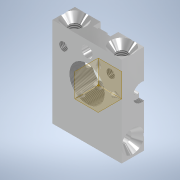
# Autodesk Inventor part: CuvetteHolderBody
Saved by Autodesk Inventor 2022 (Build 260153000, 153)
## iProperties
Created: 2021-04-01
Part Number: CuvetteHolderBody
Material: Aluminum 6061
Document SubType Name: Modeling
Designer: wilso
Density: 2.7 g/cm^3
Appearance: Aluminum - Flat
Author: wilso
Autodesk Inventor part; units mm, degrees
ref_plane "YZ Plane" through (0, 0, 0) normal (1, 0, 0) x (0, 1, 0)
ref_plane "XZ Plane" through (0, 0, 0) normal (0, 1, 0) x (-1, 0, 0)
ref_plane "XY Plane" through (0, 0, 0) normal (0, 0, 1) x (1, 0, 0)
sketch "Sketch1" plane through (0, 0, 0) normal (0, 1, 0) x (-1, 0, 0)
  line L0 (0, 0) -> (50, 0)
  line L1 (50, 0) -> (50, -16.15)
  line L2 (50, -16.15) -> (0, -16.15)
  line L3 (0, -16.15) -> (0, 0)
  dimension "d0" = 50
  dimension "d1" = 16.15
  constraints: 8 end point, 2 parallel, 1 horizontal, 1 perpendicular
  measures "d0" distance of L1.end L2.end
  measures "d1" distance of L0.end L1.end
extrude "Extrusion1" add sketch "Sketch1" along normal blind 65
sketch "Sketch2" plane through (0, 65, 0) normal (0, 1, 0) x (1, 0, 0)
  line L0 (-50, 0) -> (0, 0) projected
  line L1 (-50, 16.15) -> (-50, 0) projected
  line L2 (0, 0) -> (0, 16.15) projected
  line L3 (0, 16.15) -> (-50, 16.15) projected
  point P0 (-42.0625, 8.075)
  point P1 (-7.9375, 8.075)
  dimension "d11" = 8.075
  dimension "d12" = 7.9375
  dimension "d13" = 8.075
  dimension "d14" = 7.9375
  dimension "d87" = 16.15
  measures "d11" distance from line of L0 point (-42.062, 8.075)
  measures "d12" distance from line of L1 point (-42.062, 8.075)
  measures "d13" distance from line of L0 point (-7.938, 8.075)
  measures "d14" distance from line of L2 point (-7.938, 8.075)
  measures "d87" distance between parallel lines of L0 L3
hole "Hole1" at (-42.0625, 65, -8.075) at (-7.9375, 65, -8.075) direction (0, -1, 0) diameter 6.35 depth 55 tip angle 118 countersink diameter 16.5 countersink angle 82
sketch "Sketch3" plane through (0, 65, 0) normal (0, 1, 0) x (1, 0, 0)
  line L0 (0, 16.15) -> (-50, 16.15) projected
  line L1 (-18.65, 16.15) -> (-18.65, 10.65)
  line L2 (-18.65, 10.65) -> (-21.825, 10.65)
  line L3 (-21.825, 10.65) -> (-21.825, 11.65)
  line L4 (-21.825, 11.65) -> (-28.175, 11.65)
  line L5 (-28.175, 11.65) -> (-28.175, 10.65)
  line L6 (-28.175, 10.65) -> (-31.35, 10.65)
  line L7 (-31.35, 10.65) -> (-31.35, 16.15)
  point P0 (0, 0)
  dimension "d15" = 5.5
  dimension "d16" = 3.175
  dimension "d17" = 1
  dimension "d18" = 3.175
  dimension "d19" = 6.35
  dimension "d21" = 18.65
  constraints: 14 end point, 6 perpendicular, 4 point on line
  measures "d15" distance of L1.start L1.end
  measures "d16" distance of L1.end L2.end
  measures "d17" distance of L2.end L3.end
  measures "d18" distance of L5.end L6.end
  measures "d19" distance of L3.end L4.end
  measures "d21" distance of L0.end L7.end
extrude "Extrusion2" cut sketch "Sketch3" against normal blind 25
sketch "Sketch4" plane through (-50, 0, 0) normal (0, 0, 1) x (1, 0, 0)
  line L0 (0, 65) -> (50, 65) projected
  line L1 (0, 0) -> (0, 65) projected
  point P0 (50, 0)
  point P1 (25, 37.5)
  dimension "d24" = 27.5
  dimension "d43" = 25
  measures "d24" distance from line of L0 point (25, 37.5)
  measures "d43" distance from line of L1 point (25, 37.5)
hole "Hole2" at (-25, 37.5, 0) direction (0, 0, -1) diameter 25.4 depth 55
thread "Thread1" size "1-32 UN" class "2B" standard "ANSI Unified Screw Threads" full length
sketch "Sketch5" plane through (0, 0, 0) normal (1, 0, 0) x (0, 0, -1)
  line L0 (0, 0) -> (16.15, 0) projected
  line L1 (0, 0) -> (0, 65) projected
  line L2 (16.15, 0) -> (16.15, 65) projected
  point P0 (8.075, 10)
  dimension "d34" = 10
  dimension "d35" = 8.075
  dimension "d88" = 16.15
  measures "d34" distance from line of L0 point (8.075, 10)
  measures "d35" distance from line of L1 point (8.075, 10)
  measures "d88" distance between parallel lines of L1 L2
hole "Hole3" at (0, 10, -8.075) direction (-1, 0, 0) diameter 6.35 depth 45 tip angle 118 countersink diameter 16.5 countersink angle 82
sketch "Sketch6" plane through (-50, 0, 0) normal (0, 0, 1) x (1, 0, 0)
  line L0 (50, 0) -> (50, 65) projected
  line L1 (0, 65) -> (50, 65) projected
  point P0 (25, 57.5)
  dimension "d44" = 25
  dimension "d45" = 7.5
  measures "d44" distance from line of L0 point (25, 57.5)
  measures "d45" distance from line of L1 point (25, 57.5)
hole "Hole4" at (-25, 57.5, 0) direction (0, 0, -1) diameter 7.9375 depth 10.15 tip angle 118
sketch "Sketch7" plane through (-50, 0, -16.15) normal (-1, 0, 0) x (0, 0, 1)
  line L0 (0, 24.8) -> (0, 48.4985) projected
  line L1 (0, 37.5) -> (1.75, 37.5)
  line L2 (16.15, 0) -> (0, 0) projected
  circle A0 centre (1.75, 37.5) radius 3.175
  circle A1 centre (1.75, 37.5) radius 6.35
  dimension "d53" = 1.75
  dimension "d69" = 37.5
  dimension "d70" = 1.75
  dimension "d71" = 6.35
  dimension "d72" = 12.7
  constraints: 2 centre point, 2 coincident, 2 end point, 1 horizontal
  measures "d53" distance of L1.start L1.end
  measures "d69" distance from line of L2 L1.end
  measures "d70" distance from line of L0 L1.end
  measures "d71" diameter of A0
  measures "d72" diameter of A1
extrude "Extrusion6" cut sketch "Sketch7" against normal blind 60 contours A0 L0 | L0 A0
extrude "Extrusion7" cut sketch "Sketch7" against normal blind 3.5
sketch "Sketch9" plane through (0, 0, 0) normal (1, 0, 0) x (0, 0, -1)
  circle A0 centre (14.4, 37.5) radius 6.35
  line L0 (16.15, 0) -> (16.15, 34.8508) projected
  line L1 (0, 0) -> (16.15, 0) projected
  dimension "d77" = 12.7
  dimension "d78" = 1.75
  dimension "d79" = 37.5
  constraints: 1 centre point
  measures "d77" diameter of A0
  measures "d78" distance from line of L0 A0.centre
  measures "d79" distance from line of L1 A0.centre
extrude "Extrusion8" cut sketch "Sketch9" against normal blind 3.5
thread "Thread3" size "1/2-32 UN" class "2B" standard "ANSI Unified Screw Threads" full length
sketch "Sketch10" plane through (0, 65, 0) normal (0, 1, 0) x (1, 0, 0)
  circle A0 centre (-42.0625, 8.075) radius 3.9688
  circle A1 centre (-7.9375, 8.075) radius 3.175 projected
  circle A2 centre (-7.9375, 8.075) radius 3.9688
  line L0 (-50, 16.15) -> (-50, 0)
  circle A3 centre (-42.0625, 8.075) radius 3.175 projected
  circle A4 centre (-7.9375, 8.075) radius 3.175 projected
  point P0 (0, 0)
  dimension "d89" = 7.9375
  dimension "d90" = 7.9375
  dimension "d116" = 7.9375
  constraints: 2 centre point, 2 concentric, 2 end point, 1 coincident
  measures "d89" diameter of A0
  measures "d90" diameter of A2
  measures "d116" distance from line of L0 A0.centre
extrude "Extrusion9" cut sketch "Sketch10" against normal blind 9.525 contours A0 | A1 | A2 | A3
thread "Thread4" size "5/16-18 UNC" class "2B" standard "ANSI Unified Screw Threads" full length
thread "Thread5" size "5/16-18 UNC" class "2B" standard "ANSI Unified Screw Threads" full length
sketch "Sketch11" plane through (0, 0, 0) normal (1, 0, 0) x (0, 0, -1)
  circle A0 centre (8.075, 10) radius 3.175 projected
  circle A1 centre (8.075, 10) radius 3.9688
  point P0 (0, 0)
  dimension "d97" = 7.9375
  constraints: 1 centre point, 1 coincident
  measures "d97" diameter of A1
extrude "Extrusion10" cut sketch "Sketch11" against normal blind 9.525 contours A0 | A1
sketch "Sketch14" plane through (-50, 0, 0) normal (0, 0, 1) x (1, 0, 0)
  line L0 (0, 43.6041) -> (0, 65) projected
  line L1 (0, 65) -> (7.9375, 65)
  line L2 (0, 65) -> (6.2473, 65) projected
  line L3 (7.9375, 65) -> (7.9375, 52.3)
  line L4 (50, 65) -> (43.7527, 65) projected
  line L5 (50, 65) -> (42.0625, 65)
  line L6 (42.0625, 65) -> (42.0625, 52.3)
  circle A0 centre (7.9375, 52.3) radius 3
  circle A1 centre (42.0625, 52.3) radius 3
  point P0 (50, 0)
  dimension "d104" = 7.9375
  dimension "d105" = 12.7
  dimension "d106" = 7.9375
  dimension "d107" = 12.7
  dimension "d108" = 6
  dimension "d109" = 6
  constraints: 8 end point, 2 centre point, 2 coincident, 2 collinear, 1 perpendicular, 1 vertical
  measures "d104" distance of L0.end L1.end
  measures "d105" distance of L1.end L3.end
  measures "d106" distance of L4.start L5.end
  measures "d107" distance of L5.end L6.end
  measures "d108" diameter of A0
  measures "d109" diameter of A1
extrude "Extrusion11" cut sketch "Sketch14" against normal blind 7.9375
thread "Thread6" size "M6x1" class "6H" standard "ANSI Metric M Profile" full length
thread "Thread7" size "M6x1" class "6H" standard "ANSI Metric M Profile" full length
thread "Thread8" size "5/16-18 UNC" class "2B" standard "ANSI Unified Screw Threads" full length
equation "\"d11\" = 0.5 * d87"
equation "\"d13\" = d11"
equation "\"d14\" = d12"
equation "\"d35\" = 0.5 * d88"
equation "\"d78\" = d70"
equation "\"d79\" = d69"
equation "\"d90\" = d89"
equation "\"d106\" = d104"
equation "\"d107\" = d105"
body "Solid1"
